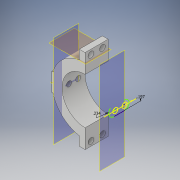
# Autodesk Inventor part: DremelHolder
Saved by Autodesk Inventor 2019 (Build 230136000, 136)
## iProperties
Created: 2019-05-13
Part Number: DremelHolder
Material: Generic
Document SubType Name: Modeling
Designer: Alex Jones
Density: 1 g/cm^3
Appearance: Default
Mass: 30.5642 g
Surface Area: 93.1195 cm^2
Volume: 30.5642 cm^3
Author: Alex Jones
Autodesk Inventor part; units mm, degrees
ref_plane "YZ Plane" through (0, 0, 0) normal (1, 0, 0) x (0, 1, 0)
ref_plane "XZ Plane" through (0, 0, 0) normal (0, 1, 0) x (-1, 0, 0)
ref_plane "XY Plane" through (0, 0, 0) normal (0, 0, 1) x (1, 0, 0)
sketch "Sketch1" plane through (0, 0, 0) normal (0, 0, 1) x (1, 0, 0)
  arc A0 (-10, -8.75) -> (-8.75, -10) centre (-8.75, -8.75) ccw projected
  line L0 (-8.75, -10) -> (-3.6, -10) projected
  line L1 (-3.6, -10) -> (-3.1, -9.5) projected
  line L2 (-3.1, -9.5) -> (-3.1, -8.4) projected
  line L3 (-3.1, -8.4) -> (-5.5, -8.4) projected
  line L4 (-5.5, -8.4) -> (-5.5, -6.466) projected
  line L5 (-5.5, -6.466) -> (-3.134, -4.1) projected
  line L6 (-3.134, -4.1) -> (3.134, -4.1) projected
  line L7 (3.134, -4.1) -> (5.5, -6.466) projected
  line L8 (5.5, -6.466) -> (5.5, -8.4) projected
  line L9 (5.5, -8.4) -> (3.1, -8.4) projected
  line L10 (3.1, -8.4) -> (3.1, -9.5) projected
  line L11 (3.1, -9.5) -> (3.6, -10) projected
  line L12 (3.6, -10) -> (8.75, -10) projected
  arc A1 (8.75, -10) -> (10, -8.75) centre (8.75, -8.75) ccw projected
  line L13 (10, -8.75) -> (10, -3.6) projected
  line L14 (10, -3.6) -> (9.5, -3.1) projected
  line L15 (9.5, -3.1) -> (8.4, -3.1) projected
  line L16 (8.4, -3.1) -> (8.4, -5.5) projected
  line L17 (8.4, -5.5) -> (6.466, -5.5) projected
  line L18 (6.466, -5.5) -> (4.1, -3.134) projected
  line L19 (4.1, -3.134) -> (4.1, 3.134) projected
  line L20 (4.1, 3.134) -> (6.466, 5.5) projected
  line L21 (6.466, 5.5) -> (8.4, 5.5) projected
  line L22 (8.4, 5.5) -> (8.4, 3.1) projected
  line L23 (8.4, 3.1) -> (9.5, 3.1) projected
  line L24 (9.5, 3.1) -> (10, 3.6) projected
  line L25 (10, 3.6) -> (10, 8.75) projected
  arc A2 (10, 8.75) -> (8.75, 10) centre (8.75, 8.75) ccw projected
  line L26 (8.75, 10) -> (3.6, 10) projected
  line L27 (3.6, 10) -> (3.1, 9.5) projected
  line L28 (3.1, 9.5) -> (3.1, 8.4) projected
  line L29 (3.1, 8.4) -> (5.5, 8.4) projected
  line L30 (5.5, 8.4) -> (5.5, 6.466) projected
  line L31 (5.5, 6.466) -> (3.134, 4.1) projected
  line L32 (3.134, 4.1) -> (-3.134, 4.1) projected
  line L33 (-3.134, 4.1) -> (-5.5, 6.466) projected
  line L34 (-5.5, 6.466) -> (-5.5, 8.4) projected
  line L35 (-5.5, 8.4) -> (-3.1, 8.4) projected
  line L36 (-3.1, 8.4) -> (-3.1, 9.5) projected
  line L37 (-3.1, 9.5) -> (-3.6, 10) projected
  line L38 (-3.6, 10) -> (-8.75, 10) projected
  arc A3 (-8.75, 10) -> (-10, 8.75) centre (-8.75, 8.75) ccw projected
  line L39 (-10, 8.75) -> (-10, 3.6) projected
  line L40 (-10, 3.6) -> (-9.5, 3.1) projected
  line L41 (-9.5, 3.1) -> (-8.4, 3.1) projected
  line L42 (-8.4, 3.1) -> (-8.4, 5.5) projected
  line L43 (-8.4, 5.5) -> (-6.466, 5.5) projected
  line L44 (-6.466, 5.5) -> (-4.1, 3.134) projected
  line L45 (-4.1, 3.134) -> (-4.1, -3.134) projected
  line L46 (-4.1, -3.134) -> (-6.466, -5.5) projected
  line L47 (-6.466, -5.5) -> (-8.4, -5.5) projected
  line L48 (-8.4, -5.5) -> (-8.4, -3.1) projected
  line L49 (-8.4, -3.1) -> (-9.5, -3.1) projected
  line L50 (-9.5, -3.1) -> (-10, -3.6) projected
  line L51 (-10, -3.6) -> (-10, -8.75) projected
  circle A4 centre (0, 0) radius 2.5 projected
  circle A5 centre (46.7, 0) radius 4.5 projected
  arc A6 (46.7103, 25.4) -> (46.7103, -25.4) centre (46.7, 0) ccw
  line L52 (10, 10) -> (16.35, 10)
  line L53 (16.35, 10) -> (16.35, -10)
  line L54 (16.35, -10) -> (10, -10)
  line L55 (10, -10) -> (10, 10)
  arc A7 (46.7103, 36.7) -> (46.7103, -36.7) centre (46.7, 0) ccw
  line L56 (46.7103, 36.7) -> (46.7103, 25.4)
  line L57 (46.7103, -25.4) -> (46.7103, -36.7)
  dimension "d0" = 50.8
  dimension "d1" = 20
  dimension "d2" = 6.35
  constraints: 12 end point, 4 point on circle, 2 centre point, 2 coincident, 2 parallel, 1 horizontal, 1 perpendicular, 1 point on line, 1 tangent
  measures "d0" diameter of A6
  measures "d1" distance of L54.end L52.start
  measures "d2" distance of L53.end L54.end
extrude "Extrusion1" add sketch "Sketch1" along normal blind 25.4 contours L13 L55 A7 L54 | L55 L25 L52 A7 | A7 L52 L53 L54 | L54 L53 L52 A7 L56 A6 L57
ref_plane "Work Plane1" through (46.7103, 36.7, 0) normal (0, 1, 0) x (0, 0, 1)
sketch "Sketch2" plane through (46.7103, 36.7, 0) normal (0, 1, 0) x (0, 0, 1)
  line L0 (0, 0) -> (25.4, 0) projected
  line L1 (25.4, -35.3216) -> (25.4, 0) projected
  line L2 (0, 0) -> (25.4, 0)
  line L3 (25.4, 0) -> (25.4, -6.35)
  line L4 (25.4, -6.35) -> (0, -6.35)
  line L5 (0, -6.35) -> (0, 0)
  point P0 (0, -46.7103)
  dimension "d6" = 6.35
  constraints: 8 end point, 2 parallel, 1 horizontal, 1 perpendicular, 1 point on line
  measures "d6" distance between parallel lines of L4 L0
extrude "Extrusion2" add sketch "Sketch2" along normal mid plane 19.05
ref_plane "Work Plane2" through (10, 0, 0) normal (0, 1, 0) x (1, 0, 0)
mirror "Mirror1" about plane through (10, 0, 0) normal (0, 1, 0) of "Extrusion2"
sketch "Sketch3" plane through (46.7103, -25.4, 25.4) normal (1, 0, 0) x (0, 0, -1)
  circle A0 centre (19.05, -15.7382) radius 3.175 projected
  circle A1 centre (6.35, -15.7382) radius 3.175 projected
  circle A2 centre (6.35, 66.5382) radius 3.175 projected
  circle A3 centre (19.05, 66.5382) radius 3.175 projected
  point P0 (25.4, 25.4)
extrude "Extrusion3" cut sketch "Sketch3" against normal through all
ref_plane "Work Plane4" through (21.3, 0, 0) normal (-1, 0, 0) x (0, -1, 0)
ref_plane "Work Plane3" through (72.1, 0, 0) normal (-1, 0, 0) x (0, -1, 0)
sketch "Sketch4" plane through (72.1, 0, 0) normal (-1, 0, 0) x (0, -1, 0)
  line L0 (0, 0) -> (0, 25.4) construction
  line L1 (-10, 25.4) -> (10, 25.4) projected
  circle A0 centre (0, 17.78) radius 2.75
  circle A1 centre (0, 7.62) radius 2.75
  line L2 (-25.4, 0) -> (25.4, 0) projected
  dimension "d13" = 5.5
  dimension "d14" = 7.62
  dimension "d15" = 7.62
  constraints: 2 centre point, 2 end point, 2 point on line, 1 equal radius, 1 midpoint
  measures "d13" diameter of A0
  measures "d14" distance from line of L1 A0.centre
  measures "d15" distance from line of L2 A1.centre
extrude "Extrusion4" cut sketch "Sketch4" along normal through all
sketch "Sketch5" plane through (72.1, 0, 0) normal (-1, 0, 0) x (0, -1, 0)
  circle A0 centre (0, 7.62) radius 2.75 projected
  line L0 (5, 19.0484) -> (5, 7.62)
  arc A1 (5, 19.0484) -> (-5, 23.3833) centre (-0.9396, 19.0484) ccw
  arc A2 (-5, 7.62) -> (5, 7.62) centre (0, 7.62) ccw
  line L1 (0, -5.08) -> (0, 30.48) projected
  point P0 (0, 0)
  dimension "d18" = 5.9396
  dimension "d20" = 5
  constraints: 5 point on circle, 2 centre point, 2 end point, 1 coincident, 1 horizontal alignment, 1 point on line, 1 tangent, 1 vertical, 2 other
  measures "d18" radius of A1
  measures "d20" distance between parallel lines of L1 L0
body "Solid1"
